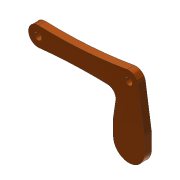
# Autodesk Inventor part: COXA_YAW_SUPPORT-LINK_BACK
Saved by Autodesk Inventor 2019.4 (Build 234330000, 330)
## iProperties
Created: 2019-10-21
Part Number: COXA_YAW_SUPPORT-LINK_BACK
Material: 一般
Document SubType Name: Modeling
Designer: y6tada
Density: 1 g/cm^3
Appearance: 滑らか - 淡いオレンジ
Author: y6tada
Autodesk Inventor part; units mm, degrees
ref_plane "YZ Plane" through (0, 0, 0) normal (1, 0, 0) x (0, 1, 0)
ref_plane "XZ Plane" through (0, 0, 0) normal (0, 1, 0) x (-1, 0, 0)
ref_plane "XY Plane" through (0, 0, 0) normal (0, 0, 1) x (1, 0, 0)
sketch "スケッチ1" plane through (0, 0, 0) normal (0, 0, 1) x (1, 0, 0)
  line L0 (0, 0) -> (0, -20) construction
  line L1 (0, -20) -> (-37.9074, -2.6507) construction
  line L2 (-37.9074, -2.6507) -> (0, 0) construction
  arc A0 (-41.6469, -1.2309) -> (-36.19, -6.2633) centre (-37.9074, -2.6507) ccw
  arc A1 (5.4905, 0.3235) -> (-1.2529, 5.3554) centre (0, 0) ccw
  arc A2 (-6.5, -23) -> (6.5, -23) centre (0, -23) ccw
  arc A3 (3.5, -17) -> (-3.5, -17) centre (0, -17) ccw
  arc A4 (-3.5, -23) -> (3.5, -23) centre (0, -23) ccw
  line L3 (-3.5, -17) -> (-3.5, -23)
  line L4 (3.5, -17) -> (3.5, -23)
  line L5 (0, -23) -> (0, -17) construction
  line L6 (5.4905, 0.3235) -> (6.4887, -16.6176)
  line L7 (6.5, -17) -> (6.5, -23)
  arc A5 (6.5, -17) -> (6.4887, -16.6176) centre (0, -17) ccw
  line L8 (-6.5, -23) -> (-6.5, -17)
  arc A6 (-1.2529, 5.3554) -> (-5.4905, 0.3235) centre (0, 0) ccw construction
  line L9 (-5.4905, 0.3235) -> (-5.7734, -4.4787) construction
  arc A7 (-6.4887, -16.6176) -> (-6.5, -17) centre (0, -17) ccw
  line L10 (-5.8372, -5.5609) -> (-6.4887, -16.6176)
  arc A8 (-5.8372, -5.5609) -> (-7.8781, -3.4437) centre (-7.8338, -5.4432) ccw
  line L11 (-40.6241, 1.4629) -> (-41.6469, -1.2309)
  arc A9 (-26, -3.8454) -> (-36.19, -6.2633) centre (-25.4454, -28.8643) ccw
  line L12 (-26, -3.8454) -> (-7.8781, -3.4437)
  arc A10 (-39.0031, 2.49) -> (-40.6241, 1.4629) centre (-39.1283, 0.8949) ccw
  arc A11 (-39.0031, 2.49) -> (-1.2529, 5.3554) centre (-29.3534, 125.4645) ccw
  line L13 (-26.133, 2.1531) -> (-8.011, 2.5548) construction
  line L14 (-39.1283, 0.8949) -> (-37.9074, -2.6507) construction
  dimension "d0" = 20
  dimension "d2" = 38
  dimension "d3" = 4
  dimension "d13" = 6
  dimension "d14" = 3.5
  dimension "d15" = 6.5
  dimension "d21" = 86
  dimension "d27" = 2
  dimension "d32" = 5.5
  dimension "d35" = 88.73
  dimension "d36" = 3.2683
  dimension "d39" = 1.6
  dimension "d40" = 26
  dimension "d41" = 6
  dimension "d42" = 105
  dimension "d43" = 3.75
  constraints: 30 end point, 26 point on circle, 24 tangent, 12 centre point, 4 coincident, 4 concentric, 4 point on line, 3 vertical, 1 equal radius, 1 midpoint, 1 parallel
  measures "d0" distance of L0.end L0.start
  measures "d2" distance of L1.end L0.start
  measures "d3" radius of A0
  measures "d13" distance of L5.start L5.end
  measures "d14" radius of A3
  measures "d15" radius of A2
  measures "d21" angle of L0 L2
  measures "d27" radius of A8
  measures "d32" radius of A1
  measures "d35" angle of L0 L12
  measures "d36" distance from line of L0.start L12
  measures "d39" radius of A10
  measures "d40" distance from line of L0 L12.start
  measures "d41" distance between parallel lines of L12 L13
  measures "d42" angle of L2 L14
  measures "d43" distance of L14.start L14.end
extrude "押し出し1" add sketch "スケッチ1" along normal blind 3
hole "穴1" at (-37.9074, -2.6507, 0) at (0, 0, 0) direction (0, 0, 1) diameter 3 end through all
sketch "スケッチ2" plane through (0, 0, 3) normal (0, 0, 1) x (1, 0, 0)
  arc A0 (3.5, -17) -> (-3.5, -17) centre (0, -17) ccw projected
  line L0 (3.5, -17) -> (3.5, -23) projected
  arc A1 (-3.5, -23) -> (3.5, -23) centre (0, -23) ccw projected
  line L1 (-3.5, -23) -> (-3.5, -17) projected
  point P0 (0, 0)
extrude "押し出し2" add sketch "スケッチ2" against normal blind 0.4
